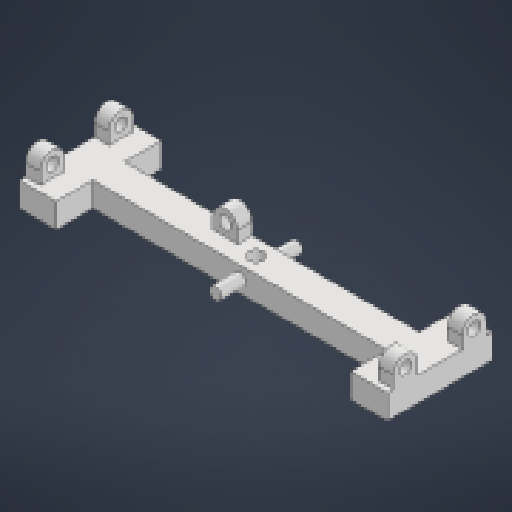
# Autodesk Inventor part: Claw Connector 2
Saved by Autodesk Inventor 2023.6 (Build 276521000, 521)
## iProperties
Created: 2026-03-05
Part Number: Claw Connector 2
Material: Generic
Document SubType Name: Modeling
Designer: user
Density: 1 g/cm^3
Appearance: Default
Author: user
Autodesk Inventor part; units mm, degrees
ref_plane "YZ Plane" through (0, 0, 0) normal (1, 0, 0) x (0, 1, 0)
ref_plane "XZ Plane" through (0, 0, 0) normal (0, 1, 0) x (-1, 0, 0)
ref_plane "XY Plane" through (0, 0, 0) normal (0, 0, 1) x (1, 0, 0)
sketch "Sketch1" plane through (0, 0, 0) normal (0, 0, 1) x (1, 0, 0)
  line L0 (-5, 5) -> (5, 5)
  line L1 (5, 5) -> (5, -5)
  line L2 (5, -5) -> (-5, -5)
  line L3 (-5, -5) -> (-5, 5)
  line L4 (-5, 5) -> (5, -5) construction
  line L5 (5, 5) -> (-5, -5) construction
  point P0 (0, 0)
  dimension "d0" = 10
  dimension "d1" = 10
  constraints: 12 end point, 2 midpoint, 2 parallel, 1 horizontal, 1 perpendicular
  measures "d0" distance between parallel lines of L2 L0
  measures "d1" distance between parallel lines of L1 L3
extrude "Extrusion1" add sketch "Sketch1" along normal blind 13
sketch "Sketch2" plane through (0, 0, 13) normal (0, 0, 1) x (1, 0, 0)
  circle A0 centre (0, 0) radius 2.35
  dimension "d4" = 4.7
  constraints: 1 centre point, 1 coincident
  measures "d4" diameter of A0
extrude "Extrusion2" add sketch "Sketch2" along normal blind 10
ref_plane "Work Plane1" through (0, 0, 6.5) normal (0, 0, 1) x (1, 0, 0)
mirror "Mirror1" about plane through (0, 0, 6.5) normal (0, 0, 1) of "Extrusion2"
sketch "Sketch3" plane through (-5, 5, 0) normal (0, 1, 0) x (1, 0, 0)
  line L0 (0, 0) -> (0, -13) projected
  line L1 (0, -6.5) -> (10, -6.5)
  line L2 (10, 0) -> (10, -13) projected
  circle A0 centre (5, -6.5) radius 3
  point P0 (5, 0)
  dimension "d7" = 6
  constraints: 3 midpoint, 2 end point, 1 centre point
  measures "d7" diameter of A0
extrude "Extrusion3" cut sketch "Sketch3" against normal through all
sketch "Sketch4" plane through (5, -5, 0) normal (1, 0, 0) x (0, 0, -1)
  line L0 (0, 0) -> (0, 10) projected
  line L1 (0, 10) -> (-13, 10) projected
  line L2 (-13, 0) -> (-13, 10) projected
  line L3 (0, 0) -> (-13, 0) projected
  point P0 (0, 5)
extrude "Extrusion4" add sketch "Sketch4" along normal blind 70
mirror "Mirror2" about plane through (0, 0, 0) normal (1, 0, 0) of "Extrusion4"
sketch "Sketch5" plane through (0, 0, 13) normal (0, 0, 1) x (1, 0, 0)
  line L0 (-75, 5) -> (75, 5) projected
  line L1 (0, 5) -> (0, -5)
  line L2 (75, -5) -> (-75, -5) projected
  line L3 (-75, 5) -> (-75, -5) projected
  line L4 (-75, -5) -> (-75, 5)
  line L5 (-60, -5) -> (-60, 5)
  line L6 (75, 5) -> (75, -5)
  line L7 (60, -5) -> (60, 5)
  point P0 (0, 0)
  dimension "d12" = 15
  constraints: 10 end point, 3 symmetric about line, 2 midpoint, 2 point on line, 1 perpendicular, 1 vertical
  measures "d12" distance between parallel lines of L5 L3
extrude "Extrusion5" add sketch "Sketch5" along normal blind 15 contours L0 L5 L2 L3 | L0 L6 L2 L7
ref_plane "Work Plane2" through (0, 0, 6.5) normal (0, 0, -1) x (-1, 0, 0)
mirror "Mirror3" about plane through (0, 0, 6.5) normal (0, 0, -1) of "Extrusion5"
sketch "Sketch6" plane through (-75, -5, 28) normal (-1, 0, 0) x (0, 0, 1)
  line L0 (-28, 10) -> (-43, 10) projected
  line L1 (-15, 10) -> (0, 10) projected
  line L2 (0, 10) -> (-43, 10) projected
  line L3 (-28, 10) -> (-43, 10)
  line L4 (-35.5, 10) -> (-35.5, 15)
  circle A0 centre (-35.5, 15) radius 2.5
  circle A1 centre (-35.5, 15) radius 5
  line L5 (-40.5, 15) -> (-40.5, 10)
  line L6 (-30.5, 15) -> (-30.5, 10)
  line L7 (-40.5, 10) -> (-30.5, 10)
  line L8 (-18.5, 0) -> (-24.5, 0) projected
  line L9 (-21.5, 0) -> (-21.5, 20.3601)
  line L10 (-15, 10) -> (0, 10)
  line L11 (-7.5, 10) -> (-7.5, 15)
  circle A2 centre (-7.5, 15) radius 2.5
  circle A3 centre (-7.5, 15) radius 5
  line L12 (-2.5, 15) -> (-2.5, 10)
  line L13 (-12.5, 15) -> (-12.5, 10)
  point P0 (-28, 5)
  dimension "d15" = 5
  dimension "d16" = 5
  dimension "d17" = 10
  constraints: 20 end point, 8 symmetric about line, 4 centre point, 4 coincident, 4 point on circle, 2 midpoint, 2 perpendicular, 2 point on line, 2 tangent, 2 vertical, 1 collinear, 1 horizontal, 2 other
  measures "d15" distance of L4.start L4.end
  measures "d16" diameter of A0
  measures "d17" diameter of A1
extrude "Extrusion6" add sketch "Sketch6" against normal blind 6
mirror "Mirror4" about plane through (0, 0, 0) normal (1, 0, 0) of "Extrusion6"
sketch "Sketch8" plane through (0, 0, 0) normal (0, 0, -1) x (-1, 0, 0)
  line L0 (3, -96.3437) -> (3, 27.6563)
  line L1 (60, 5) -> (-60, 5) projected
  line L2 (3, 5) -> (8, 5)
  line L3 (8, 5) -> (8, 10)
  circle A0 centre (13, 10) radius 5
  line L4 (60, 5) -> (-60, 5) projected
  line L5 (18, 10) -> (18, 5)
  circle A1 centre (13, 10) radius 2.5
  point P0 (0, 0)
  dimension "d22" = 10
  dimension "d20" = 5
  dimension "d21" = 5
  dimension "d23" = 5
  constraints: 8 end point, 4 point on line, 3 vertical, 1 centre point, 1 coincident, 1 horizontal, 1 perpendicular, 5 other
  measures "d20" distance of L2.start L2.end
  measures "d21" distance of L2.end L3.end
  measures "d23" diameter of A1
extrude "Extrusion7" add sketch "Sketch8" against normal blind 6
body "Solid1"
